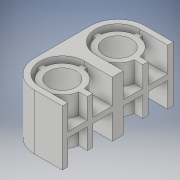
# Autodesk Inventor part: straight_beam_inner_part
Saved by Autodesk Inventor 2019 (Build 230136000, 136)
## iProperties
Created: 2019-01-31
Part Number: straight_beam_inner_part
Material: Generic
Document SubType Name: Modeling
Designer: Varga Daniel
Density: 1 g/cm^3
Appearance: Default
Author: Varga Daniel
Autodesk Inventor part; units mm, degrees
ref_plane "YZ Plane" through (0, 0, 0) normal (1, 0, 0) x (0, 1, 0)
ref_plane "XZ Plane" through (0, 0, 0) normal (0, 1, 0) x (-1, 0, 0)
ref_plane "XY Plane" through (0, 0, 0) normal (0, 0, 1) x (1, 0, 0)
derived "Base_part.ipt"
sketch "Sketch1" plane through (0, 0, 0) normal (0, 1, 0) x (-1, 0, 0)
  line L0 (5, 0) -> (25, 0)
  line L1 (30, 5) -> (30, 25)
  line L2 (25, 30) -> (5, 30)
  line L3 (0, 25) -> (0, 5)
  line L4 (5, 29) -> (25, 29)
  line L5 (29, 25) -> (29, 5)
  line L6 (25, 1) -> (5, 1)
  line L7 (1, 5) -> (1, 25)
  circle A0 centre (5, 5) radius 2.5
  circle A1 centre (5, 5) radius 3.5
  arc A2 (25, 0) -> (30, 5) centre (25, 5) ccw
  arc A3 (30, 25) -> (25, 30) centre (25, 25) ccw
  arc A4 (5, 30) -> (0, 25) centre (5, 25) ccw
  arc A5 (0, 5) -> (5, 0) centre (5, 5) ccw
  arc A6 (1, 5) -> (5, 1) centre (5, 5) ccw
  arc A7 (5, 29) -> (1, 25) centre (5, 25) ccw
  arc A8 (29, 25) -> (25, 29) centre (25, 25) ccw
  arc A9 (25, 1) -> (29, 5) centre (25, 5) ccw
  line L8 (49.1041, 15) -> (-27.081, 15) construction
  line L9 (31.1478, 10) -> (-2.4877, 10) construction
  line L10 (-2.8604, 5) -> (35.495, 5) construction
  line L11 (5, -2.5736) -> (5, 36.7522) construction
  line L12 (15, -1.4978) -> (15, 34.8784) construction
  line L13 (1.5359, 5.5) -> (1, 5.5)
  line L14 (1.5359, 4.5) -> (1.0314, 4.5)
  line L15 (28.9686, 4.5) -> (8.4641, 4.5)
  line L16 (29, 5.5) -> (8.4641, 5.5)
  line L17 (4.5, 1.5359) -> (4.5, 1.0314)
  line L18 (5.5, 1.5359) -> (5.5, 1)
  line L19 (29, 10.5) -> (1, 10.5)
  line L20 (29, 9.5) -> (1, 9.5)
  line L21 (4.5, 28.9686) -> (4.5, 10.5)
  line L22 (4.5, 9.5) -> (4.5, 8.4641)
  line L23 (5.5, 29) -> (5.5, 10.5)
  line L24 (5.5, 9.5) -> (5.5, 8.4641)
  point P0 (0, 0)
  point P1 (30, 30)
  point P2 (0, 30)
  point P3 (5, 25)
sketch "Sketch3" plane through (0, 0, 0) normal (0, 1, 0) x (-1, 0, 0)
  circle A0 centre (5, 5) radius 2.5 construction
  circle A1 centre (5, 5) radius 3.5 construction
  circle A2 centre (5, 5) radius 2.5
  arc A3 (1.5359, 5.5) -> (8.4641, 5.5) centre (5, 5) ccw
  line L0 (0.3508, 5) -> (13.598, 5) construction
  line L1 (5, 15) -> (5, -1.7484) construction
  line L2 (0, 20) -> (0, 14.5)
  line L3 (5, 1) -> (4.5, 1)
  line L4 (0, 1) -> (0, 0)
  line L5 (0, 0) -> (5, 0)
  line L6 (0, 0) -> (0, 1)
  line L7 (1.5359, 5.5) -> (0, 5.5)
  line L8 (0, 5.5) -> (0, 4.5)
  line L9 (0, 4.5) -> (1.5359, 4.5)
  line L10 (4.5, 1.5359) -> (4.5, 1)
  line L11 (0, 9) -> (0, 10)
  line L12 (5, 20) -> (0, 20)
  line L13 (10, 10) -> (0, 10) construction
  line L14 (9, 9) -> (5, 9)
  line L15 (9, 11) -> (5.5, 11)
  line L16 (10, 15) -> (0, 15) construction
  line L17 (5, 19) -> (0, 19)
  circle A4 centre (5, 15) radius 2.5
  arc A5 (8.4641, 14.5) -> (1.5359, 14.5) centre (5, 15) ccw
  line L18 (1.5359, 14.5) -> (0, 14.5)
  line L19 (1.5359, 15.5) -> (0, 15.5)
  line L20 (9, 9) -> (0, 9)
  arc A6 (10, 15) -> (5, 20) centre (5, 15) ccw
  line L21 (10, 5) -> (10, 15)
  line L22 (9, 15) -> (9, 14.5)
  arc A7 (9, 15) -> (5, 19) centre (5, 15) ccw
  arc A8 (5, 0) -> (10, 5) centre (5, 5) ccw
  arc A9 (5, 1) -> (9, 5) centre (5, 5) ccw
  line L23 (5.5, 1.5359) -> (5.5, 1.0314)
  line L24 (9, 5.5) -> (8.4641, 5.5)
  line L25 (8.9686, 4.5) -> (8.4641, 4.5)
  line L26 (8.9686, 15.5) -> (8.4641, 15.5)
  line L27 (9, 14.5) -> (8.4641, 14.5)
  line L28 (9, 14.5) -> (9, 11)
  line L29 (9, 9) -> (5.5, 9)
  line L30 (4.5, 9) -> (0, 9)
  line L31 (5, 11) -> (0, 11)
  arc A10 (5.5, 11.5359) -> (8.4641, 14.5) centre (5, 15) ccw
  arc A11 (4.5, 8.4641) -> (1.5359, 5.5) centre (5, 5) ccw
  arc A12 (5.5, 8.4641) -> (4.5, 8.4641) centre (5, 5) ccw
  arc A13 (8.4641, 5.5) -> (5.5, 8.4641) centre (5, 5) ccw
  arc A14 (4.5, 11.5359) -> (5.5, 11.5359) centre (5, 15) ccw
  line L32 (5.5, 9) -> (5.5, 8.4641)
  line L33 (4.5, 9) -> (4.5, 8.4641)
  line L34 (4.5, 1) -> (0, 1)
  line L35 (0, 1) -> (0, 9)
  line L36 (4.5, 11) -> (0, 11)
  line L37 (4.5, 11) -> (0, 11)
  line L38 (5.5, 11.5359) -> (5.5, 11)
  line L39 (4.5, 11.5359) -> (4.5, 11)
  arc A15 (1.5359, 14.5) -> (4.5, 11.5359) centre (5, 15) ccw
  line L40 (9, 11) -> (9, 5)
  line L41 (5.5, 11) -> (4.5, 11)
  arc A16 (5.5, 11.5359) -> (8.4641, 14.5) centre (5, 15) ccw
  arc A17 (8.4641, 14.5) -> (1.5359, 14.5) centre (5, 15) ccw
  line L42 (0, 11) -> (0, 5.5)
  line L43 (0, 14.5) -> (0, 11)
  line L44 (5.5, 18.9686) -> (5.5, 18.4641)
  line L45 (4.5, 19) -> (4.5, 18.4641)
  line L46 (2, 11) -> (0, 11)
  point P0 (0, 0)
  point P1 (5, 15)
  dimension "d4" = 1
  dimension "d21" = 2
  dimension "d25" = 1
  dimension "d26" = 5
  dimension "d27" = 7
  dimension "d28" = 7
  dimension "d29" = 5
  dimension "d30" = 1
  dimension "d43" = 1
  dimension "d44" = 1
  dimension "d45" = 1
  dimension "d63" = 10
  constraints: 94 end point, 59 point on circle, 37 point on line, 19 parallel, 16 centre point, 13 collinear, 10 tangent, 9 perpendicular, 6 coincident, 6 vertical, 4 horizontal, 4 midpoint, 2 concentric, 6 other
  measures "d4" distance between parallel lines of L3 L5
  measures "d21" distance between parallel lines of L14 L15
  measures "d25" distance between parallel lines of L12 L17
  measures "d26" diameter of A0
  measures "d27" diameter of A1
  measures "d28" diameter of A5
  measures "d29" diameter of A4
  measures "d30" distance between parallel lines of L19 L18
  measures "d43" distance between parallel lines of L22 L21
  measures "d44" distance between parallel lines of L10 L23
  measures "d45" distance between parallel lines of L9 L7
  measures "d63" distance between parallel lines of L16 L0
ref_plane "Work Plane2" through (0, 0, 1) normal (0, -1, 0) x (0, 0, 1)
extrude "Extrusion13" add sketch "Sketch3" along normal blind 5 contours L3 A9 L40 L28 L22 A7 L17 L2 L12 A6 L21 A8 L5 L4 L34
extrude "Extrusion14" add sketch "Sketch3" against normal blind 5 contours L3 A9 L40 L28 L22 A7 L17 L2 L12 A6 L21 A8 L5 L4 L34
extrude "Extrusion15" add sketch "Sketch3" along normal blind 0.5 contours L7 L35 L20 L33 A11 | A3 L10 L34 L35 L9 | L32 L14 L40 L24 A13 | A3 L25 A9 L23 | L43 L18 A15 L39 L31 | L15 L38 A10 L27 L28 | L2 L17 L45 A5 L19 | L26 A5 L44 A7
extrude "Extrusion16" add sketch "Sketch3" against normal blind 0.5 contours L7 L35 L20 L33 A11 | A3 L10 L34 L35 L9 | L32 L14 L40 L24 A13 | A3 L25 A9 L23 | L43 L18 A15 L39 L31 | L15 L38 A10 L27 L28 | L2 L17 L45 A5 L19 | L26 A5 L44 A7
extrude "Extrusion17" add sketch "Sketch3" along normal blind 5 contours L11 L42 L31 L41 L15 L40 L14 L20
extrude "Extrusion18" add sketch "Sketch3" against normal blind 5 contours L11 L42 L31 L41 L15 L40 L14 L20
extrude "Extrusion19" add sketch "Sketch3" along normal blind 4.2 contours A11 A12 A13 A3 | A3 L9 L8 L7 | L33 L20 L14 L32 A12 | A3 L23 A9 L3 L10 | L24 L40 A9 L25 A3 | L2 L19 A5 L18 | L39 A14 L38 L41 L31 | A5 A10 A14 A15 | L27 A5 L26 A7 L22 | L17 A7 L44 A5 L45
extrude "Extrusion20" add sketch "Sketch3" against normal blind 4.2 contours A11 A12 A13 A3 | A3 L9 L8 L7 | L33 L20 L14 L32 A12 | A3 L23 A9 L3 L10 | L24 L40 A9 L25 A3 | L2 L19 A5 L18 | L39 A14 L38 L41 L31 | A5 A10 A14 A15 | L27 A5 L26 A7 L22 | L17 A7 L44 A5 L45
fillet "Fillet1" radius 4 4 edges at (-9, -2.75, 9) (-9, -2.75, 11) (-9, 2.75, 9) (-9, 2.75, 11)
equation "\"d4\" = Wall_thickness"
equation "\"d21\" = 2 * Wall_thickness"
equation "\"d25\" = Wall_thickness"
equation "\"d28\" = d27"
equation "\"d29\" = d26"
equation "\"d30\" = Inner_route_thickness"
equation "\"d43\" = Wall_thickness"
equation "\"d44\" = Inner_route_thickness"
equation "\"d45\" = Inner_route_thickness"
equation "\"d46\" = 0.5 * Overall_height"
equation "\"d48\" = 0.5 * Overall_height"
equation "\"d50\" = 0.5 * Inner_thickness"
equation "\"d52\" = 0.5 * Inner_thickness"
equation "\"d54\" = 0.5 * Overall_height"
equation "\"d56\" = 0.5 * Overall_height"
equation "\"d58\" = 0.5 * Hole_height"
equation "\"d60\" = 0.5 * Hole_height"
equation "\"Wall_thickness\" = 1"
equation "\"Inner_route_thickness\" = 1"
equation "\"Overall_height\" = 10"
equation "\"Inner_thickness\" = 1"
equation "\"Hole_height\" = 8.4"
body "Solid3"
